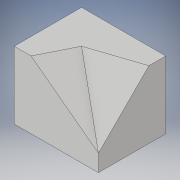
# Autodesk Inventor part: 零件24
Saved by Autodesk Inventor 2019 (Build 230136000, 136)
## iProperties
Created: 2020-09-18
Part Number: 零件24
Material: 一般
Document SubType Name: Modeling
Designer: jay
Density: 1 g/cm^3
Appearance: 預設
Author: jay
Autodesk Inventor part; units mm, degrees
ref_plane "YZ Plane" through (0, 0, 0) normal (1, 0, 0) x (0, 1, 0)
sketch "草圖1" plane through (0, 0, 0) normal (0, 0, 1) x (1, 0, 0)
  line L0 (0, 0) -> (50, 0)
  line L1 (50, 0) -> (50, 40)
  line L2 (50, 40) -> (0, 40)
  line L3 (0, 40) -> (0, 0)
  dimension "d0" = 50
  dimension "d1" = 40
  constraints: 8 end point, 2 parallel, 1 horizontal, 1 perpendicular
  measures "d0" distance of L1.end L2.end
  measures "d1" distance of L0.end L1.end
extrude "擠出1" add sketch "草圖1" along normal blind 40
sketch "草圖7" plane through (0, 40, 0) normal (0, 1, 0) x (1, 0, 0)
  line L0 (0, -40) -> (50, -40) projected
  line L1 (0, 0) -> (0, -40) projected
  line L2 (50, 0) -> (0, 0) projected
  line L3 (50, 0) -> (50, -40) projected
  point P0 (50, -10)
  point P1 (20, -20)
  point P2 (10, -40)
  dimension "d13" = 10
  dimension "d14" = 20
  dimension "d15" = 20
  dimension "d16" = 10
  constraints: 2 point on line
  measures "d13" distance from line of L1 point (10, -40)
  measures "d14" distance from line of L1 point (20, -20)
  measures "d15" distance from line of L2 point (20, -20)
  measures "d16" distance from line of L2 point (50, -10)
sketch "草圖8" plane through (0, 0, 40) normal (0, 0, 1) x (1, 0, 0)
  line L0 (50, 0) -> (50, 40) projected
  line L1 (0, 0) -> (50, 0) projected
  line L2 (50, 0) -> (50, 40) projected
  line L3 (50, 40) -> (0, 40) projected
  line L4 (0, 40) -> (0, 0) projected
  point P0 (50, 10)
  dimension "d17" = 10
  constraints: 1 point on line
  measures "d17" distance from line of L1 point (50, 10)
ref_plane "工作平面3" through (20, 40, 20) normal (0.5747, 0.7663, 0.2873) x (-0.4472, 0, 0.8944)
sketch "草圖9" plane through (20, 40, 20) normal (0.5747, 0.7663, 0.2873) x (-0.4472, 0, 0.8944)
  line L0 (0, 0) -> (4.4721, 46.6905)
  line L1 (4.4721, 46.6905) -> (22.3607, 0)
  line L2 (22.3607, 0) -> (0, 0)
  point P0 (-8.9443, 5.1402)
  constraints: 6 end point, 1 horizontal
extrude "擠出4" cut sketch "草圖9" along normal blind 40
ref_plane "工作平面4" through (50, 40, 10) normal (0.2294, 0.6882, 0.6882) x (-0.9487, 0, 0.3162)
sketch "草圖11" plane through (50, 40, 10) normal (0.2294, 0.6882, 0.6882) x (-0.9487, 0, 0.3162)
  line L0 (31.6228, 0) -> (9.4868, 41.3521)
  line L1 (9.4868, 41.3521) -> (0, 0)
  line L2 (0, 0) -> (31.6228, 0)
  point P0 (44.2719, 11.6076)
  constraints: 6 end point, 1 horizontal
extrude "擠出5" cut sketch "草圖11" along normal blind 40
